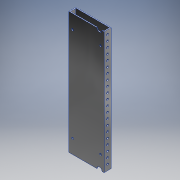
# Autodesk Inventor part: Mid
Saved by Autodesk Inventor 2019.4 (Build 234330000, 330)
## iProperties
Created: 2019-11-04
Part Number: Mid
Material: Aluminum 6061
Document SubType Name: Modeling
Designer: Mark
Density: 2.7 g/cm^3
Appearance: Aluminum - Flat
Mass: 561.254 g
Surface Area: 2088 cm^2
Volume: 207.872 cm^3
Author: Mark
Autodesk Inventor part; units mm, degrees
ref_plane "YZ Plane" through (0, 0, 0) normal (1, 0, 0) x (0, 1, 0)
ref_plane "XZ Plane" through (0, 0, 0) normal (0, 1, 0) x (-1, 0, 0)
ref_plane "XY Plane" through (0, 0, 0) normal (0, 0, 1) x (1, 0, 0)
sketch "Sketch1" plane through (0, 0, 0) normal (0, 1, 0) x (-1, 0, 0)
  line L0 (50, -10) -> (-50, -10)
  line L1 (-50, -10) -> (-50, 10)
  line L2 (-50, 10) -> (50, 10)
  line L3 (50, 10) -> (50, -10)
  line L4 (50, -10) -> (-50, 10) construction
  line L5 (-50, -10) -> (50, 10) construction
  line L6 (48, -8) -> (-48, -8)
  line L7 (-48, -8) -> (-48, 8)
  line L8 (-48, 8) -> (48, 8)
  line L9 (48, 8) -> (48, -8)
  line L10 (48, -8) -> (-48, 8) construction
  line L11 (-48, -8) -> (48, 8) construction
  point P0 (0, 0)
  dimension "d2" = 100
  dimension "d3" = 20
  dimension "d4" = 96
  dimension "d5" = 16
  constraints: 24 end point, 4 midpoint, 4 parallel, 2 horizontal, 2 perpendicular
  measures "d2" distance of L1.end L2.end
  measures "d3" distance of L0.end L1.end
  measures "d4" distance of L7.end L8.end
  measures "d5" distance of L6.end L7.end
extrude "Extrusion1" add sketch "Sketch1" along normal blind 348
sketch "Sketch2" plane through (-50, 0, 10) normal (0, 0, 1) x (1, 0, 0)
  circle A0 centre (10, 40) radius 2.75
  circle A1 centre (90, 40) radius 2.75
  circle A2 centre (10, 308) radius 2.75
  circle A3 centre (90, 308) radius 2.75
  line L0 (0, 348) -> (100, 348) projected
  line L1 (0, 0) -> (0, 348) projected
  line L2 (100, 0) -> (100, 348) projected
  line L3 (100, 0) -> (0, 0) projected
  point P0 (50, 0)
  dimension "d8" = 5.5
  dimension "d9" = 5.5
  dimension "d10" = 5.5
  dimension "d11" = 5.5
  dimension "d12" = 40
  dimension "d13" = 10
  dimension "d14" = 10
  dimension "d15" = 40
  dimension "d16" = 40
  dimension "d17" = 10
  dimension "d18" = 40
  dimension "d19" = 10
  constraints: 4 centre point
  measures "d8" diameter of A0
  measures "d9" diameter of A1
  measures "d10" diameter of A2
  measures "d11" diameter of A3
  measures "d12" distance from line of L0 A2.centre
  measures "d13" distance from line of L1 A2.centre
  measures "d14" distance from line of L2 A3.centre
  measures "d15" distance from line of L0 A3.centre
  measures "d16" distance from line of L3 A0.centre
  measures "d17" distance from line of L1 A0.centre
  measures "d18" distance from line of L3 A1.centre
  measures "d19" distance from line of L2 A1.centre
extrude "Extrusion2" cut sketch "Sketch2" against normal through all contours A0 | A1 | A2 | A3
sketch "Sketch3" plane through (-50, 0, -10) normal (-1, 0, 0) x (0, 0, 1)
  circle A0 centre (10, 16) radius 2.75
  line L0 (10, 16) -> (10, 0) construction
  line L1 (0, 0) -> (0, 348) projected
  circle A1 centre (10, 32) radius 2.75
  circle A2 centre (10, 48) radius 2.75
  circle A3 centre (10, 64) radius 2.75
  circle A4 centre (10, 80) radius 2.75
  circle A5 centre (10, 96) radius 2.75
  circle A6 centre (10, 112) radius 2.75
  circle A7 centre (10, 128) radius 2.75
  circle A8 centre (10, 144) radius 2.75
  circle A9 centre (10, 160) radius 2.75
  circle A10 centre (10, 176) radius 2.75
  circle A11 centre (10, 192) radius 2.75
  circle A12 centre (10, 208) radius 2.75
  circle A13 centre (10, 224) radius 2.75
  circle A14 centre (10, 240) radius 2.75
  circle A15 centre (10, 256) radius 2.75
  circle A16 centre (10, 272) radius 2.75
  circle A17 centre (10, 288) radius 2.75
  circle A18 centre (10, 304) radius 2.75
  circle A19 centre (10, 320) radius 2.75
  circle A20 centre (10, 336) radius 2.75
  circle A21 centre (10, 352) radius 2.75
  circle A22 centre (10, 368) radius 2.75
  circle A23 centre (10, 384) radius 2.75
  circle A24 centre (10, 400) radius 2.75
  circle A25 centre (10, 416) radius 2.75
  circle A26 centre (10, 432) radius 2.75
  dimension "d22" = 5.5
  dimension "d23" = 16
  dimension "d26" = 16
  constraints: 27 centre point, 2 end point, 2 vertical, 52 other
  measures "d22" diameter of A0
  measures "d23" distance of L0.start L0.end
  measures "d26" distance of L0.start A1.centre
extrude "Extrusion3" cut sketch "Sketch3" against normal through all
sketch "Sketch4" plane through (-50, 0, 10) normal (0, 0, 1) x (1, 0, 0)
  line L0 (0, 348) -> (100, 348) projected
  circle A0 centre (87, 348) radius 7.5
  line L1 (2, 348) -> (98, 348) projected
  line L2 (100, 0) -> (0, 0) projected
  circle A1 centre (87, 0) radius 7.5
  line L3 (100, 0) -> (100, 348) projected
  point P0 (50, 0)
  dimension "d33" = 15
  dimension "d35" = 15
  dimension "d36" = 13
  dimension "d37" = 13
  constraints: 3 point on line, 2 centre point
  measures "d33" diameter of A0
  measures "d35" diameter of A1
  measures "d36" distance from line of L3 A0.centre
  measures "d37" distance from line of L3 A1.centre
extrude "Extrusion4" cut sketch "Sketch4" against normal blind 10
body "Solid1"
